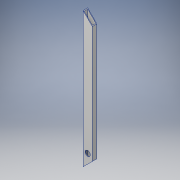
# Autodesk Inventor part: AngleBrace.ver2-1111-2020
Saved by Autodesk Inventor 2018 (Build 220112000, 112)
## iProperties
Created: 2020-01-19
Part Number: AngleBrace.ver2-1111-2020
Material: Aluminum 6061
Document SubType Name: Modeling
Designer: JMHal
Density: 2.7 g/cm^3
Appearance: Aluminum - Flat
Author: JMHal
Autodesk Inventor part; units mm, degrees
ref_plane "YZ Plane" through (0, 0, 0) normal (1, 0, 0) x (0, 1, 0)
ref_plane "XZ Plane" through (0, 0, 0) normal (0, 1, 0) x (-1, 0, 0)
ref_plane "XY Plane" through (0, 0, 0) normal (0, 0, 1) x (1, 0, 0)
sketch "Sketch1" plane through (0, 0, 0) normal (0, 1, 0) x (-1, 0, 0)
  line L0 (0, 0) -> (50.8, 0)
  line L1 (50.8, 0) -> (50.8, -25.4)
  line L2 (50.8, -25.4) -> (0, -25.4)
  line L3 (0, -25.4) -> (0, 0)
  line L4 (47.625, -22.225) -> (47.625, -3.175)
  line L5 (47.625, -3.175) -> (3.175, -3.175)
  line L6 (3.175, -3.175) -> (3.175, -22.225)
  line L7 (3.175, -22.225) -> (47.625, -22.225)
  dimension "d0" = 50.8
  dimension "d1" = 25.4
  dimension "d2" = 3.175
  constraints: 16 end point, 4 parallel, 2 perpendicular, 1 horizontal, 3 other
  measures "d0" distance of L1.end L2.end
  measures "d1" distance of L0.end L1.end
  measures "d2" distance between parallel lines of L1 L4
extrude "Extrusion1" add sketch "Sketch1" along normal blind 886.206
sketch "Sketch2" plane through (-50.8, 0, 0) normal (0, 0, 1) x (1, 0, 0)
  line L0 (50.8, 0) -> (0, 0) projected
  line L1 (50.8, 0) -> (50.8, 886.206) projected
  line L2 (0, 886.206) -> (50.8, 886.206) projected
  line L3 (0, 0) -> (0, 886.206) projected
  line L4 (0, 0) -> (50.8, 0) projected
  line L5 (50.8, 0) -> (0, 56.4191)
  line L6 (0, 56.4191) -> (50.8, 56.4191)
  line L7 (50.8, 56.4191) -> (50.8, 0)
  line L8 (50.8, 0) -> (0, 0)
  line L9 (0, 0) -> (0, 56.4191)
  line L10 (0, 56.4191) -> (50.8, 0)
  line L11 (0, 56.4191) -> (21.859, 0)
  line L12 (47.625, 0) -> (3.175, 0) projected
  dimension "d5" = 48
  constraints: 14 end point, 2 parallel, 2 point on line, 1 horizontal, 1 perpendicular
  measures "d5" angle of L5 L0
extrude "Extrusion2" cut sketch "Sketch2" against normal blind 914.4 contours L0 L11 L5 | L11 L0 L3
sketch "Sketch3" plane through (-50.8, 886.206, 0) normal (0, 0, 1) x (1, 0, 0)
  line L0 (0, -829.7869) -> (50.8, -886.206) projected
  line L1 (50.8, -886.206) -> (50.8, 0) projected
  line L2 (0, 0) -> (50.8, 0) projected
  line L3 (0, -829.7869) -> (0, 0) projected
  line L4 (0, -829.7869) -> (50.8, -886.206) projected
  line L5 (0, -829.7869) -> (50.8, -778.9869)
  line L6 (50.8, -886.206) -> (50.8, 0) projected
  line L7 (0, -829.7869) -> (0, 0) projected
  line L8 (50.8, -886.206) -> (0, -886.206)
  line L9 (0, -886.206) -> (0, -923.3654)
  line L10 (0, -923.3654) -> (50.8, -923.3654)
  line L11 (50.8, -923.3654) -> (50.8, -886.206)
  dimension "d8" = 93
  constraints: 10 end point, 4 point on line, 2 parallel, 1 horizontal, 1 perpendicular
  measures "d8" angle of L0 L5
extrude "Extrusion3" cut sketch "Sketch3" against normal blind 25.4 contours L5 L1 L0
sketch "Sketch4" plane through (-50.8, 886.206, 0) normal (0, 0, 1) x (1, 0, 0)
  line L0 (0, -829.7869) -> (50.8, -778.9869) projected
  line L1 (50.8, -778.9869) -> (50.8, 0) projected
  line L2 (0, 0) -> (50.8, 0) projected
  line L3 (0, -829.7869) -> (0, 0) projected
  line L4 (0, 0) -> (50.8, 0) projected
  line L5 (0, 0) -> (50.8, 0)
  line L6 (50.8, 0) -> (50.8, -221.7928)
  line L7 (50.8, -221.7928) -> (0, -221.7928)
  line L8 (0, -221.7928) -> (0, 0)
  line L9 (0, -829.7869) -> (0, 0) projected
  line L10 (0, 0) -> (50.8, -50.8)
  line L11 (50.8, 0) -> (0, 0)
  line L12 (0, 0) -> (0, -56.4191)
  line L13 (0, -56.4191) -> (50.8, -56.4191)
  line L14 (50.8, -56.4191) -> (50.8, 0)
  point P0 (50.8, -886.206)
  dimension "d11" = 221.7928
  dimension "d12" = 45
  dimension "d13" = 56.4191
  constraints: 18 end point, 4 parallel, 3 point on line, 2 horizontal, 2 perpendicular
  measures "d11" distance between parallel lines of L7 L2
  measures "d12" angle of L2 L10
  measures "d13" distance between parallel lines of L13 L2
extrude "Extrusion4" cut sketch "Sketch4" against normal blind 25.4 contours L2 L1 L10
sketch "Sketch8" plane through (-50.8, 56.4191, 0) normal (0, 0, 1) x (1, 0, 0)
  line L0 (50.8, 778.9869) -> (0, 829.7869) projected
  line L1 (0, 0) -> (0, 829.7869) projected
  line L2 (0, 0) -> (50.8, 50.8) projected
  line L3 (50.8, 50.8) -> (50.8, 778.9869) projected
  line L4 (0, 797.6016) -> (50.8, 746.8016)
  point P0 (50.8, -56.4191)
  dimension "d24" = 22.7584
  constraints: 2 end point, 2 point on line
  measures "d24" distance between parallel lines of L0 L4
extrude "Extrusion8" cut sketch "Sketch8" against normal blind 25.4 contours L3 L4 L1 L0
sketch "Sketch9" plane through (-50.8, 56.4191, 0) normal (0, 0, 1) x (1, 0, 0)
  line L0 (50.8, 746.8016) -> (0, 797.6016) projected
  line L1 (0, 0) -> (0, 797.6016) projected
  line L2 (0, 0) -> (50.8, 50.8) projected
  line L3 (50.8, 50.8) -> (50.8, 746.8016) projected
  line L4 (0, 0) -> (0, 797.6016) projected
  line L5 (0, 58.228) -> (50.8, 109.028)
  line L6 (50.8, 50.8) -> (50.8, 746.8016) projected
  line L7 (0, 0) -> (50.8, 50.8) projected
  point P0 (50.8, -56.4191)
  dimension "d27" = 41.1734
  constraints: 2 end point, 2 point on line, 1 parallel
  measures "d27" distance between parallel lines of L5 L2
extrude "Extrusion9" cut sketch "Sketch9" against normal blind 25.4 contours L3 L2 L1 L5
sketch "Sketch10" plane through (-50.8, 114.6471, 0) normal (0, 0, 1) x (1, 0, 0)
  line L0 (0, 0) -> (50.8, 50.8) projected
  line L1 (50.8, 50.8) -> (50.8, 688.5737) projected
  line L2 (50.8, 688.5737) -> (0, 739.3737) projected
  line L3 (0, 0) -> (0, 739.3737) projected
  point P0 (50.8, -114.6471)
  point P1 (25.4, 76.2)
hole "Hole1" at (-25.4, 190.8471, 0) direction (0, 0, -1) diameter 28.575 end through all
body "Solid1"
